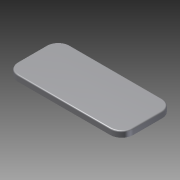
# Autodesk Inventor part: Placa
Saved by Autodesk Inventor 2011 SP2 (Build 150309200, 309)
## iProperties
Created: 2023-03-20
Part Number: Placa
Document SubType Name: Modeling
Designer: utilizator
Density: 1 g/cm^3
Author: utilizator
Autodesk Inventor part; units mm, degrees
ref_plane "YZ Plane" through (0, 0, 0) normal (1, 0, 0) x (0, 1, 0)
ref_plane "XZ Plane" through (0, 0, 0) normal (0, 1, 0) x (-1, 0, 0)
ref_plane "XY Plane" through (0, 0, 0) normal (0, 0, 1) x (1, 0, 0)
sketch "Sketch1" plane through (0, 0, 0) normal (0, 0, 1) x (1, 0, 0)
  line L0 (-145.799, 0) -> (145.799, 0) projected
  line L1 (0, -68.799) -> (0, 68.799) projected
  line L2 (-80, 45) -> (80, 45)
  line L3 (100, 25) -> (100, -25)
  line L4 (80, -45) -> (-80, -45)
  line L5 (-100, -25) -> (-100, 25)
  arc A0 (-80, 45) -> (-100, 25) centre (-80, 25) ccw
  arc A1 (100, 25) -> (80, 45) centre (80, 25) ccw
  arc A2 (80, -45) -> (100, -25) centre (80, -25) ccw
  arc A3 (-100, -25) -> (-80, -45) centre (-80, -25) ccw
  point P0 (0, 0)
  point P1 (-100, 45)
  point P2 (100, -45)
  point P3 (-100, -45)
  point P4 (0, 45)
  dimension "d0" = 200
  dimension "d1" = 90
  dimension "d2" = 45
  dimension "d3" = 20
  constraints: 8 end point, 8 point on circle, 8 tangent, 6 point on line, 4 centre point, 3 equal radius, 2 parallel, 1 horizontal, 1 midpoint, 1 perpendicular, 1 vertical alignment
  measures "d0" distance of point (100, -45) point (-100, -45)
  measures "d1" distance of point (-100, -45) point (-100, 45)
  measures "d2" distance between parallel lines of L4 L0
  measures "d3" radius of A0
extrude "Extrusion1" add sketch "Sketch1" along normal blind 10
fillet "Fillet1" radius 2 8 edges at (-94.1421, -39.1421, 10) (-100, 0, 10) (-94.1421, 39.1421, 10) (0, 45, 10) (94.1421, 39.1421, 10) (100, 0, 10) (94.1421, -39.1421, 10) (0, -45, 10)
body "Solid1"
